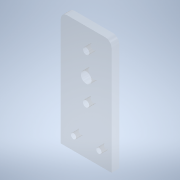
# Autodesk Inventor part: BaseC_5
Saved by Autodesk Inventor 2021 (Build 250183000, 183)
## iProperties
Created: 2023-10-20
Part Number: BaseC_5
Material: PMMA Plastic
Document SubType Name: Modeling
Designer: user
Density: 1.23982 g/cm^3
Appearance: Polycarbonate - Clear
Mass: 25.78 g
Surface Area: 89.7239 cm^2
Volume: 20.7933 cm^3
Author: user
Autodesk Inventor part; units mm, degrees
ref_plane "YZ Plane" through (0, 0, 0) normal (1, 0, 0) x (0, 1, 0)
ref_plane "XZ Plane" through (0, 0, 0) normal (0, 1, 0) x (-1, 0, 0)
ref_plane "XY Plane" through (0, 0, 0) normal (0, 0, 1) x (1, 0, 0)
sketch "Sketch1" plane through (0, 0, 0) normal (0, 0, 1) x (1, 0, 0)
  line L0 (40, 4.4544) -> (40, 94.4544)
  line L1 (40, 94.4544) -> (0, 94.4544)
  line L2 (0, 94.4544) -> (0, 4.4544)
  circle A0 centre (20, 59.4544) radius 4.25
  circle A1 centre (10, 14.4544) radius 2.1
  circle A2 centre (30, 14.4544) radius 2.1
  circle A3 centre (19.982, 77.4544) radius 2.5
  circle A4 centre (19.8755, 41.4544) radius 2.5
  line L3 (0, 4.4544) -> (40, 4.4544)
  point P0 (0, 0)
  dimension "d4" = 40
  dimension "d5" = 90
  dimension "d7" = 8.5
  dimension "d8" = 35
  dimension "d9" = 20
  dimension "d11" = 90
  dimension "d19" = 10
  dimension "d21" = 4.2
  dimension "d22" = 10
  dimension "d24" = 4.2
  constraints: 8 end point, 5 centre point, 2 coincident, 1 horizontal, 1 parallel
  measures "d4" distance of L1.end L0.end
  measures "d5" distance of L0.end L0.start
  measures "d7" diameter of A0
  measures "d8" distance from line of A0.centre L1
  measures "d9" distance from line of L2 A0.centre
  measures "d11" distance of L1.end L2.end
  measures "d19" distance from line of L2 point (10, 14.454)
  measures "d21" diameter of A1
  measures "d22" distance from line of L0 point (30, 14.454)
  measures "d24" diameter of A2
extrude "Extrusion1" add sketch "Sketch1" along normal blind 6
fillet "Fillet1" radius 5 2 edges at (0, 94.4544, 3) (40, 94.4544, 3)
equation "\"d9\" = 0.5 * d4"
equation "\"d22\" = d19"
equation "\"d24\" = d21"
body "Solid1"
